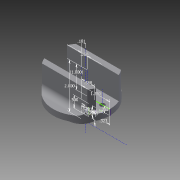
# Autodesk Inventor part: denso-1in-square-tube coupler
Saved by Autodesk Inventor 2015 (Build 190159000, 159)
## iProperties
Created: 2015-02-04
Part Number: denso-1in-square-tube coupler
Material: Generic
Document SubType Name: Modeling
Designer: sethbattis
Density: 1 g/cm^3
Appearance: Default
Author: sethbattis
Autodesk Inventor part; units mm, degrees
ref_plane "YZ Plane" through (0, 0, 0) normal (1, 0, 0) x (0, 1, 0)
ref_plane "XZ Plane" through (0, 0, 0) normal (0, 1, 0) x (-1, 0, 0)
ref_plane "XY Plane" through (0, 0, 0) normal (0, 0, 1) x (1, 0, 0)
sketch "Sketch1" plane through (0, 0, 0) normal (0, 0, 1) x (1, 0, 0)
  line L0 (0, 0) -> (0, 50.8) construction
  line L1 (0, 0) -> (50.8, 0) construction
  line L2 (0, 50.8) -> (6.35, 50.8) construction
  line L3 (6.35, 50.8) -> (6.35, 0) construction
  line L4 (0, 25.4) -> (14.9225, 25.4) construction
  line L5 (0, 18.9992) -> (31.75, 18.9992) construction
  line L6 (31.75, 18.9992) -> (31.75, 25.4)
  line L7 (14.9225, 25.4) -> (31.75, 25.4)
  line L8 (0, 9.5479) -> (15.8115, 9.5479) construction
  line L9 (31.75, 18.9992) -> (15.875, 18.9992)
  line L10 (15.875, 18.9992) -> (15.875, 6.2992)
  line L11 (15.875, 18.9992) -> (28.575, 18.9992) construction
  line L12 (0, 22.1996) -> (31.75, 22.1996) construction
  line L13 (0, 6.2992) -> (8.2867, 6.2992) construction
  line L14 (8.2867, 6.2992) -> (15.875, 6.2992)
  line L15 (8.2867, 6.2992) -> (8.2867, 18.9992)
  line L16 (23.5585, 11.9908) -> (23.5585, 41.3472) construction
  line L17 (4.5974, 71.0633) -> (4.5974, -11.3243) construction
  line L18 (8.2867, 18.9992) -> (4.5974, 18.9992)
  line L19 (4.5974, 25.4) -> (6.35, 25.4)
  line L20 (4.5974, 25.4) -> (4.5974, 18.9992)
  line L21 (6.35, 25.4) -> (14.9225, 25.4)
  dimension "d2" = 50.8
  dimension "d3" = 90
  dimension "d4" = 6.35
  dimension "d6" = 14.9225
  dimension "d9" = 31.75
  dimension "d11" = 6.4008
  dimension "d12" = 15.8115
  dimension "d13" = 12.7
  dimension "d14" = 90
  dimension "d15" = 8.2867
  dimension "d28" = 8.1915
  dimension "d55" = 4.5974
  dimension "d56" = 12.7
  dimension "d57" = 25.4
  constraints: 45 end point, 10 point on line, 7 perpendicular, 6 horizontal, 5 midpoint, 4 vertical, 2 collinear, 1 horizontal alignment, 1 parallel
  measures "d2" distance of L0.start L0.end
  measures "d3" angle of L1 L0
  measures "d4" distance of L0.end L2.end
  measures "d6" distance of L4.start L4.end
  measures "d9" distance of L5.start L5.end
  measures "d11" distance of L5.end L6.end
  measures "d12" distance of L8.start L8.end
  measures "d13" distance of L9.end L10.end
  measures "d14" angle of L10 L11
  measures "d15" distance of L13.start L13.end
  measures "d28" distance between parallel lines of L6 L16
  measures "d55" distance between parallel lines of L0 L17
  measures "d56" distance of L13.end L15.end
  measures "d57" distance of L2.end L19.end
revolve "Revolution1" add sketch "Sketch1" angle 360 about axis through (0, 0, 0) along (0, 1, 0)
fillet "Fillet2" radius 3.175 1 edges at (-15.875, 18.9992, 0)
hole "Hole2" at (23.4944, 25.4, -0.034) direction (0, -1, 0) diameter 5.3975 end through all
pattern_circular "Circular Pattern1" count 2 over 360 about axis through (0, 22.1996, 0) along (0, -1, 0) of "Hole2"
sketch "Sketch2" plane through (0, 6.2992, 0) normal (0, -1, 0) x (1, 0, 0)
  circle A0 centre (0, 0) radius 8.2867 construction
  line L0 (-2.2055, 7.9879) -> (-2.2121, 9.8928)
  circle A1 centre (0, 0) radius 10.1371 construction
  line L1 (2.1506, 8.0028) -> (2.144, 9.9078)
  line L2 (-2.2055, 7.9879) -> (2.1506, 8.0028) construction
  arc A2 (2.144, 9.9078) -> (-2.2121, 9.8928) centre (0, 0) ccw
  arc A3 (2.1506, 8.0028) -> (-2.2055, 7.9879) centre (0, 0) ccw
  dimension "d43" = 1.905
  dimension "d44" = 4.3561
  constraints: 8 point on circle, 6 end point, 3 centre point, 2 coincident, 1 concentric, 1 parallel, 1 perpendicular
  measures "d43" distance of L0.start L0.end
  measures "d44" distance of L0.start L1.start
extrude "Extrusion1" cut sketch "Sketch2" against normal blind 12.7
pattern_circular "Circular Pattern2" count 6 over 360 about axis through (0, 12.6492, 0) along (0, -1, 0) of "Extrusion1"
sketch "Sketch4" plane through (0, 25.4, 0) normal (0, 1, 0) x (1, 0, 0)
  line L0 (-29.0994, 12.7) -> (29.0994, 12.7)
  line L1 (29.0994, -12.7) -> (-29.0994, -12.7)
  circle A0 centre (0, 0) radius 31.75 construction
  line L2 (-31.75, 0) -> (31.75, 0) construction
  line L3 (-25.4, 19.05) -> (25.4, 19.05)
  line L4 (-25.4, -19.05) -> (25.4, -19.05)
  arc A1 (-25.4, 19.05) -> (-29.0994, 12.7) centre (0, 0) ccw
  arc A2 (29.0994, 12.7) -> (25.4, 19.05) centre (0, 0) ccw
  arc A3 (-29.0994, -12.7) -> (-25.4, -19.05) centre (0, 0) ccw
  arc A4 (25.4, -19.05) -> (29.0994, -12.7) centre (0, 0) ccw
  dimension "d58" = 25.4
  dimension "wallThickness" = 6.35
  dimension "d60" = 6.35
  constraints: 10 end point, 8 point on circle, 4 centre point, 4 horizontal, 2 parallel, 12 other
  measures "d58" distance of L0.end L1.start
  measures "wallThickness" distance between parallel lines of L0 L3
  measures "d60" distance between parallel lines of L4 L1
extrude "Extrusion3" add sketch "Sketch4" along normal blind 25.4
fillet "Fillet3" radius 6.35 2 edges at (0, 25.4, 19.05) (0, 25.4, -19.05)
body "Solid1"
